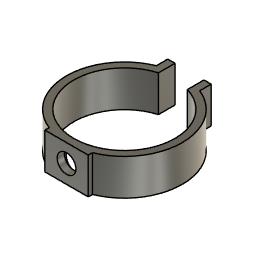
Halterung-Loch v0 (Autodesk Fusion 360 design; units mm, degrees)
Autodesk Fusion 360 part; units mm, degrees
sketch "Skizze1" plane through (0, 0, 0) normal (0, 0, 1) x (1, 0, 0)
  circle A0 centre (0, 0) radius 35
  circle A1 centre (0, 0) radius 40
  line L0 (10, 30) -> (-10, 30)
  line L1 (-10, 30) -> (-10, 45)
  line L2 (-10, 45) -> (10, 45)
  line L3 (10, 45) -> (10, 30)
  line L4 (15, 35) -> (10, 35)
  line L5 (10, 35) -> (10, 45)
  line L6 (10, 45) -> (15, 45)
  line L7 (15, 45) -> (15, 35)
  line L8 (-10, 35) -> (-15, 35)
  line L9 (-15, 35) -> (-15, 45)
  line L10 (-15, 45) -> (-10, 45)
  line L11 (-10, 45) -> (-10, 35)
  line L12 (-15, -35) -> (15, -35)
  line L13 (15, -35) -> (15, -40)
  line L14 (15, -40) -> (-15, -40)
  line L15 (-15, -40) -> (-15, -35)
  dimension "d1" = 70
  dimension "d2" = 80
  constraint coincident A0.centre A1.centre
  constraint horizontal L0
  constraint vertical L1
  constraint horizontal L2
  constraint vertical L3
  constraint horizontal L4
  constraint vertical L5
  constraint horizontal L6
  constraint vertical L7
  constraint horizontal L8
  constraint vertical L9
  constraint horizontal L10
  constraint vertical L11
  constraint coincident L1 L8.start
  constraint horizontal L12
  constraint vertical L13
  constraint horizontal L14
  constraint vertical L15
  measures "d1" diameter of A0
  measures "d2" diameter of A1
extrude "Extrusion1" add sketch "Skizze1" along normal blind 25 contours A0 A1 L3 L4 L7 L12 L13 | A0 A1 L1 L8 L9 L12 L15 | A1 L12 L13 L15 | A1 L3 L4 L5 L7 | A1 L1 L8 L9 L11 | A1 L3 L5 L6 L7 | A1 L14 L15 | A1 L13 L14 | A1 L1 L9 L10 L11
hole "Bohrung1" at (0, -40, 12.5) direction (0, 1, 0) diameter 13 depth 5 tip angle 118
